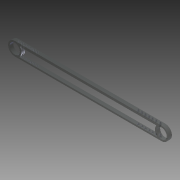
# Autodesk Inventor part: chainparts
Saved by Autodesk Inventor 2011 (Build 150239000, 239)
## iProperties
Created: 2013-01-19
Part Number: chainparts
Document SubType Name: Modeling
Designer: Danny
Density: 1 g/cm^3
Author: Danny
Autodesk Inventor part; units mm, degrees
ref_plane "YZ Plane" through (0, 0, 0) normal (1, 0, 0) x (0, 1, 0)
ref_plane "XZ Plane" through (0, 0, 0) normal (0, 1, 0) x (-1, 0, 0)
ref_plane "XY Plane" through (0, 0, 0) normal (0, 0, 1) x (1, 0, 0)
sketch "Sketch1" plane through (0, 0, 0) normal (0, 0, 1) x (1, 0, 0)
  circle A0 centre (-520.7, 0) radius 18.292
  arc A1 (-520.7, 23.8855) -> (-520.7, -23.8855) centre (-520.7, 0) ccw
  circle A2 centre (0, 0) radius 18.292
  arc A3 (-18.292, 15.3597) -> (-15.3597, -18.292) centre (0, 0) ccw
  line L0 (-520.7, 23.8855) -> (0, 23.8855)
  line L1 (0, -23.8855) -> (-520.7, -23.8855)
  line L2 (-502.408, 15.3597) -> (-18.292, 15.3597)
  line L3 (-15.3597, -18.292) -> (-505.3403, -18.292)
  arc A4 (-505.3403, -18.292) -> (-502.408, 15.3597) centre (-520.7, 0) ccw
  arc A5 (0, -23.8855) -> (0, 23.8855) centre (0, 0) ccw
  constraints: 10 point on circle, 8 end point, 6 centre point, 6 tangent, 3 coincident, 2 parallel
extrude "Extrusion1" add sketch "Sketch1" along normal blind 12.7
hole "Hole1" at (-511.8427, 23.8855, 6.35) direction (0, -1, 0) diameter 6.35 end through all
hole "Hole2" at (-500.1982, 23.8855, 5.969) direction (0, -1, 0) diameter 6.35 end through all
hole "Hole3" at (-487.7816, 23.8855, 6.3246) direction (0, -1, 0) diameter 6.35 end through all
hole "Hole4" at (-477.4438, 23.8855, 5.9436) direction (0, -1, 0) diameter 6.35 end through all
hole "Hole5" at (-466.5726, 23.8855, 5.969) direction (0, -1, 0) diameter 6.35 depth 25.4 tip angle 118
hole "Hole6" at (-457.4032, 23.8855, 6.0706) direction (0, -1, 0) diameter 6.35 end through all
hole "Hole7" at (-467.1387, -18.292, 6.35) direction (0, -1, 0) diameter 6.35 depth 25.4 tip angle 118
hole "Hole8" at (-446.1256, 23.8855, 6.8072) direction (0, -1, 0) diameter 6.35 end through all
hole "Hole9" at (-26.2382, 23.8855, 5.6642) direction (0, -1, 0) diameter 6.35 end through all
hole "Hole10" at (-39.0144, 23.8855, 6.35) direction (0, -1, 0) diameter 6.35 end through all
hole "Hole11" at (-50.8508, 23.8855, 6.35) direction (0, -1, 0) diameter 6.35 end through all
hole "Hole12" at (-64.3636, 23.8855, 6.35) direction (0, -1, 0) diameter 6.35 end through all
hole "Hole13" at (-76.581, 23.8855, 5.6896) direction (0, -1, 0) diameter 6.35 end through all
hole "Hole14" at (-89.1794, 23.8855, 5.969) direction (0, -1, 0) diameter 6.35 end through all
hole "Hole15" at (-11.43, 23.8855, 5.3848) direction (0, -1, 0) diameter 6.35 end through all
body "Solid1"
